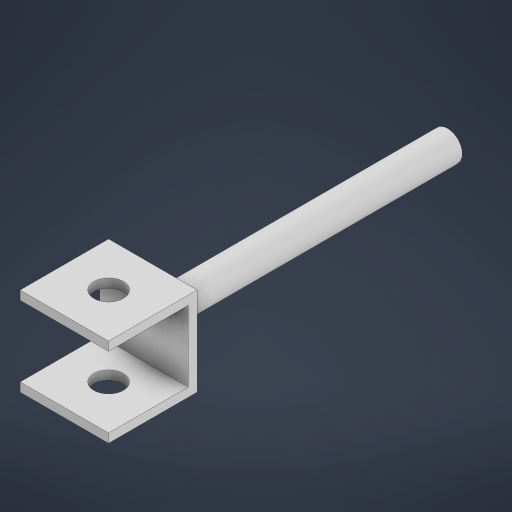
# Autodesk Inventor part: Tensioner
Saved by Autodesk Inventor 2023 (Build 270158000, 158)
## iProperties
Created: 2023-11-07
Part Number: Tensioner
Material: Generic
Document SubType Name: Modeling
Designer: Abhinav
Density: 1 g/cm^3
Appearance: Default
Author: Abhinav
Autodesk Inventor part; units mm, degrees
ref_plane "YZ Plane" through (0, 0, 0) normal (1, 0, 0) x (0, 1, 0)
ref_plane "XZ Plane" through (0, 0, 0) normal (0, 1, 0) x (-1, 0, 0)
ref_plane "XY Plane" through (0, 0, 0) normal (0, 0, 1) x (1, 0, 0)
sketch "Sketch1" plane through (0, 0, 0) normal (1, 0, 0) x (0, 1, 0)
  line L0 (12, 1.5) -> (-12, 1.5)
  line L1 (-15, 1.5) -> (-15, -1.5)
  line L2 (-15, -1.5) -> (15, -1.5)
  line L3 (15, -1.5) -> (15, 1.5)
  line L4 (15, 1.5) -> (-15, -1.5) construction
  line L5 (-15, 1.5) -> (15, -1.5) construction
  line L6 (15, -1.5) -> (12, -1.5)
  line L7 (12, 28.5) -> (15, 28.5)
  line L8 (15, 28.5) -> (15, -1.5)
  line L9 (-15, -1.5) -> (-12, -1.5)
  line L10 (-12, 28.5) -> (-15, 28.5)
  line L11 (-15, 28.5) -> (-15, -1.5)
  line L12 (12, -1.5) -> (12, -1.2)
  line L13 (12, 1.2) -> (12, 28.5)
  line L14 (-12, -1.5) -> (-12, -1.2)
  line L15 (-12, 1.2) -> (-12, 28.5)
  point P0 (0, 0)
  dimension "d0" = 30
  dimension "d1" = 3
  dimension "d2" = 3
  dimension "d3" = 30
  dimension "d4" = 3
  dimension "d5" = 30
  constraints: 32 end point, 8 parallel, 6 point on line, 5 perpendicular, 3 horizontal, 2 midpoint
  measures "d0" distance of L2.end L1.end
  measures "d1" distance of L1.end L1.start
  measures "d2" distance of L7.start L7.end
  measures "d3" distance of L6.end L7.start
  measures "d4" distance of L10.end L10.start
  measures "d5" distance of L10.start L9.end
extrude "Extrusion1" add sketch "Sketch1" along normal blind 30
sketch "Sketch2" plane through (0, 15, 28.5) normal (0, 1, 0) x (1, 0, 0)
  line L0 (0, 30) -> (30, 30) construction
  line L1 (0, 0) -> (30, 30) construction
  circle A0 centre (15, 15) radius 5
  point P0 (0, 28.5)
  dimension "d8" = 10
  constraints: 2 end point, 1 centre point, 1 midpoint
  measures "d8" diameter of A0
extrude "Extrusion2" cut sketch "Sketch2" against normal blind 30
sketch "Sketch3" plane through (0, -15, -1.5) normal (0, 0, -1) x (-1, 0, 0)
  line L0 (0, 0) -> (-30, 0) construction
  line L1 (0, 30) -> (-30, 30) construction
  line L2 (-30, 0) -> (0, 30) construction
  circle A0 centre (-15, 15) radius 5
  point P0 (0, 15)
  dimension "d11" = 10
  constraints: 2 end point, 1 centre point, 1 midpoint
  measures "d11" diameter of A0
extrude "Extrusion3" add sketch "Sketch3" along normal blind 100
body "Solid1"
